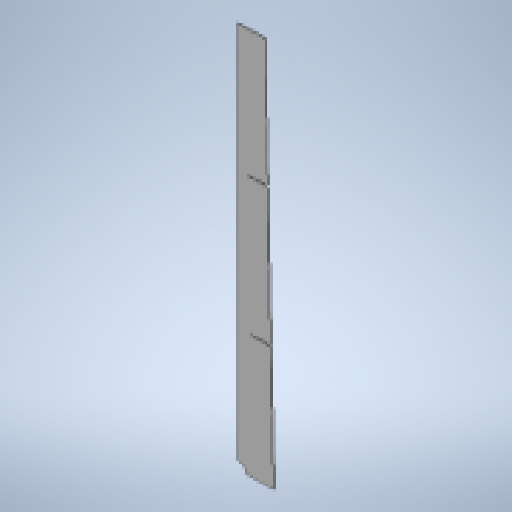
# Autodesk Inventor part: GBK 3311 central third rib_CPY1
Saved by Autodesk Inventor 2026.2 (Build 302298000, 298)
## iProperties
Created: 2026-04-17
Part Number: GBK 3311 central third rib_CPY1
Material: Steel
Document SubType Name: Sheet Metal
Designer: pokla
Mass: 5375.64 g
Surface Area: 3562.08 cm^2
Volume: 684.794 cm^3
Density: 7.85 g/cm^3
Flat Pattern Width: 13.2265 cm
Flat Pattern Length: 140.963 cm
Flat Pattern Area: 1864.45 cm^2
Sheet Metal Rule: Default
Sheet Metal Width: 132,265 mm
Sheet Metal Length: 1409,631 mm
Sheet Metal Area: 186445,444 mm^2
Appearance: Default
Stock Number: 3311
Author: pokla
Autodesk Inventor part; units mm, degrees
ref_plane "YZ Plane" through (0, 0, 0) normal (1, 0, 0) x (0, 1, 0)
ref_plane "XZ Plane" through (0, 0, 0) normal (0, 1, 0) x (-1, 0, 0)
ref_plane "XY Plane" through (0, 0, 0) normal (0, 0, 1) x (1, 0, 0)
sketch "Sketch1" plane through (0, 0, 0) normal (0, 0, 1) x (1, 0, 0)
  line L0 (0, 0) -> (0, 4368.8557)
  line L1 (0, 4368.8557) -> (100, 4368.8557)
  line L2 (100, 4368.8557) -> (200, 0)
  line L3 (200, 0) -> (0, 0)
  circle A0 centre (0, 0) radius 30
  line L4 (0, 1479.6125) -> (166.1327, 1479.6125)
  line L5 (0, 2959.2249) -> (132.2654, 2959.2249)
  circle A1 centre (0, 1479.6125) radius 30
  circle A2 centre (0, 2959.2249) radius 30
  line L6 (190.7298, 405) -> (120.7298, 405)
  line L7 (120.7298, 405) -> (120.7298, 410)
  line L8 (120.7298, 410) -> (190.7298, 410)
  line L9 (190.7298, 410) -> (190.7298, 405)
  line L10 (109.2882, 909.8691) -> (179.2882, 909.8691)
  line L11 (179.2882, 904.8691) -> (109.2882, 904.8691)
  line L12 (109.2882, 904.8691) -> (109.2882, 909.8691)
  line L13 (179.2882, 909.8691) -> (179.2882, 904.8691)
  line L14 (97.8465, 1409.7381) -> (167.8465, 1409.7381)
  line L15 (167.8465, 1404.7381) -> (97.8465, 1404.7381)
  line L16 (97.8465, 1404.7381) -> (97.8465, 1409.7381)
  line L17 (167.8465, 1409.7381) -> (167.8465, 1404.7381)
  line L18 (86.4049, 1909.6072) -> (156.4049, 1909.6072)
  line L19 (156.4049, 1904.6072) -> (86.4049, 1904.6072)
  line L20 (86.4049, 1904.6072) -> (86.4049, 1909.6072)
  line L21 (156.4049, 1909.6072) -> (156.4049, 1904.6072)
  line L22 (74.9632, 2409.4763) -> (144.9632, 2409.4763)
  line L23 (144.9632, 2404.4763) -> (74.9632, 2404.4763)
  line L24 (74.9632, 2404.4763) -> (74.9632, 2409.4763)
  line L25 (144.9632, 2409.4763) -> (144.9632, 2404.4763)
  line L26 (63.5216, 2909.3454) -> (133.5216, 2909.3454)
  line L27 (133.5216, 2904.3454) -> (63.5216, 2904.3454)
  line L28 (63.5216, 2904.3454) -> (63.5216, 2909.3454)
  line L29 (133.5216, 2909.3454) -> (133.5216, 2904.3454)
  line L30 (52.08, 3409.2144) -> (122.08, 3409.2144)
  line L31 (122.08, 3404.2144) -> (52.08, 3404.2144)
  line L32 (52.08, 3404.2144) -> (52.08, 3409.2144)
  line L33 (122.08, 3409.2144) -> (122.08, 3404.2144)
  line L34 (40.6383, 3909.0835) -> (110.6383, 3909.0835)
  line L35 (110.6383, 3904.0835) -> (40.6383, 3904.0835)
  line L36 (40.6383, 3904.0835) -> (40.6383, 3909.0835)
  line L37 (110.6383, 3909.0835) -> (110.6383, 3904.0835)
  line L38 (0, 1629.6125) -> (162.6993, 1629.6125)
  line L39 (0, 3079.2249) -> (129.5187, 3079.2249)
  point P0 (30, 2959.2249)
  point P1 (0, 2929.2249)
  point P2 (0, 1509.6125)
  point P3 (0, 1449.6125)
  point P4 (0, 30)
  point P5 (30, 0)
  point P6 (190.6154, 410)
  point P7 (179.2882, 904.8691)
  point P8 (179.1737, 909.8691)
  point P9 (167.8465, 1404.7381)
  point P10 (167.7321, 1409.7381)
  point P11 (30, 1479.6125)
  point P12 (156.4049, 1904.6072)
  point P13 (156.2904, 1909.6072)
  point P14 (144.9632, 2404.4763)
  point P15 (144.8488, 2409.4763)
  point P16 (133.5216, 2904.3454)
  point P17 (133.4072, 2909.3454)
  point P18 (0, 2989.2249)
  point P19 (122.08, 3404.2144)
  point P20 (121.9655, 3409.2144)
  point P21 (110.6383, 3904.0835)
  point P22 (110.5239, 3909.0835)
  dimension "d65" = 100
  dimension "d67" = 200
  dimension "d68" = 60
  dimension "d69" = 1480
  dimension "d70" = 1480
  dimension "d71" = 1410
  dimension "d72" = 5
  dimension "d73" = 70
  dimension "d74" = 410
  dimension "d77" = 500
  dimension "d82" = 120
  dimension "d83" = 150
  measures "d65" distance of L0.end L1.end
  measures "d67" distance of L3.start L0.start
  measures "d68" diameter of A0
  measures "d69" distance of L4.end L3.start
  measures "d70" distance of L4.end L5.end
  measures "d71" distance of L1.end L5.end
  measures "d72" distance of L6.end L7.end
  measures "d73" distance of L6.start L6.end
  measures "d74" distance between parallel lines of L3 L8
  measures "d77" distance of L7.end L10.start
  measures "d82" distance between parallel lines of L5 L39
  measures "d83" distance between parallel lines of L38 L4
extrude "Plate3" add sketch "Sketch1" along normal blind 4 contours L39 L2 L5 A2 L0 | L0 L1 L2 L34 L36 L35 L30 L32 L31 L39
chamfer "Corner Chamfer2" distance 3 angle 45 4 edges at (122.08, 3404.2144, 2) (121.9655, 3409.2144, 2) (110.6383, 3904.0835, 2) (110.5239, 3909.0835, 2)
equation "\"BendRadius\" = Thickness"
equation "\"BendReliefWidth\" = Thickness"
equation "\"BendReliefDepth\" = 0.5 * Thickness"
equation "\"CornerReliefSize\" = 4 * Thickness"
equation "\"MinimumRemnant\" = 2 * Thickness"
equation "\"TransitionRadius\" = BendRadius"
equation "\"JacobiRadiusSize\" = BendRadius"
equation "\"GapSize\" = Thickness"
equation "\"Thickness\" = 4"
body "Solid2"
